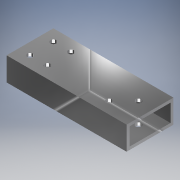
# Autodesk Inventor part: 15102898-16-P-0801
Saved by Autodesk Inventor 2017 (Build 210142000, 142)
## iProperties
Created: 2016-10-10
Part Number: 15102898-16-P-0801
Material: Aluminum 6061
Document SubType Name: Modeling
Designer: gus
Density: 2.7 g/cm^3
Appearance: Aluminum - Flat
Author: gus
Autodesk Inventor part; units mm, degrees
ref_plane "YZ Plane" through (0, 0, 0) normal (1, 0, 0) x (0, 1, 0)
ref_plane "XZ Plane" through (0, 0, 0) normal (0, 1, 0) x (-1, 0, 0)
ref_plane "XY Plane" through (0, 0, 0) normal (0, 0, 1) x (1, 0, 0)
sketch "Sketch1" plane through (0, 0, 0) normal (1, 0, 0) x (0, 1, 0)
  line L0 (0, 0) -> (25.4, 0)
  line L1 (25.4, 0) -> (25.4, -50.8)
  line L2 (25.4, -50.8) -> (0, -50.8)
  line L3 (0, -50.8) -> (0, 0)
  line L4 (22.225, -47.625) -> (22.225, -3.175)
  line L5 (22.225, -3.175) -> (3.175, -3.175)
  line L6 (3.175, -3.175) -> (3.175, -47.625)
  line L7 (3.175, -47.625) -> (22.225, -47.625)
  dimension "d0" = 25.4
  dimension "d1" = 50.8
  dimension "d2" = 3.175
  constraints: 16 end point, 4 parallel, 2 perpendicular, 1 horizontal, 3 other
  measures "d0" distance of L1.end L2.end
  measures "d1" distance of L0.end L1.end
  measures "d2" distance between parallel lines of L1 L4
extrude "Extrusion1" add sketch "Sketch1" along normal blind 130.175
sketch "Sketch2" plane through (0, 0, -50.8) normal (0, -1, 0) x (1, 0, 0)
  circle A0 centre (114.3, 22.225) radius 3.175
  circle A1 centre (98.425, 38.1) radius 3.175
  line L0 (130.175, 50.8) -> (130.175, 0) projected
  line L1 (0, 50.8) -> (130.175, 50.8) projected
  circle A2 centre (9.525, 12.7) radius 3.175
  circle A3 centre (9.525, 38.1) radius 3.175
  circle A4 centre (28.575, 12.7) radius 3.175
  circle A5 centre (28.575, 38.1) radius 3.175
  line L2 (0, 0) -> (0, 50.8) projected
  line L3 (0, 0) -> (130.175, 0) projected
  dimension "d5" = 6.35
  dimension "d6" = 6.35
  dimension "d7" = 31.75
  dimension "d8" = 15.875
  dimension "d9" = 28.575
  dimension "d10" = 12.7
  dimension "d13" = 6.35
  dimension "d14" = 6.35
  dimension "d15" = 6.35
  dimension "d16" = 6.35
  dimension "d17" = 12.7
  dimension "d18" = 12.7
  dimension "d19" = 9.525
  dimension "d20" = 9.525
  dimension "d21" = 12.7
  dimension "d22" = 12.7
  dimension "d23" = 25.4
  dimension "d24" = 28.575
  constraints: 6 centre point
  measures "d5" diameter of A0
  measures "d6" diameter of A1
  measures "d7" distance from line of L0 A1.centre
  measures "d8" distance from line of L0 A0.centre
  measures "d9" distance from line of L1 A0.centre
  measures "d10" distance from line of L1 A1.centre
  measures "d13" diameter of A2
  measures "d14" diameter of A3
  measures "d15" diameter of A4
  measures "d16" diameter of A5
  measures "d17" distance from line of L1 A5.centre
  measures "d18" distance from line of L1 A3.centre
  measures "d19" distance from line of L2 A2.centre
  measures "d20" distance from line of L2 A3.centre
  measures "d21" distance from line of L3 A2.centre
  measures "d22" distance from line of L3 A4.centre
  measures "d23" distance of A4.centre A5.centre
  measures "d24" distance from line of L2 A5.centre
extrude "Extrusion2" cut sketch "Sketch2" against normal blind 25.4 contours A0 | A1 | A2 | A3 | A4 | A5
body "Solid1"
